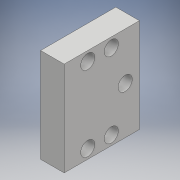
# Autodesk Inventor part: base_topPart
Saved by Autodesk Inventor 2018 (Build 220112000, 112)
## iProperties
Created: 2019-10-09
Part Number: base_topPart
Material: 一般
Document SubType Name: Modeling
Designer: Eiji Nishizawa
Density: 1 g/cm^3
Appearance: 既定
Author: Eiji Nishizawa
Autodesk Inventor part; units mm, degrees
ref_plane "YZ Plane" through (0, 0, 0) normal (1, 0, 0) x (0, 1, 0)
ref_plane "XZ Plane" through (0, 0, 0) normal (0, 1, 0) x (-1, 0, 0)
ref_plane "XY Plane" through (0, 0, 0) normal (0, 0, 1) x (1, 0, 0)
sketch "スケッチ1" plane through (0, 0, 0) normal (1, 0, 0) x (0, 1, 0)
  line L0 (-7.9816, 10) -> (7.9816, 10)
  line L1 (7.9816, 10) -> (7.9816, -10)
  line L2 (7.9816, -10) -> (-7.9816, -10)
  line L3 (-7.9816, -10) -> (-7.9816, 10)
  line L4 (-7.9816, 10) -> (7.9816, -10) construction
  line L5 (7.9816, 10) -> (-7.9816, -10) construction
  circle A0 centre (-2.9816, 8) radius 1.5
  circle A1 centre (2.0184, 8) radius 1.5
  circle A2 centre (2.0184, -8) radius 1.5
  circle A3 centre (-2.9816, -8) radius 1.5
  circle A4 centre (4.9684, 0) radius 1.5
  point P0 (0, 0)
  dimension "d0" = 3
  dimension "d1" = 3
  dimension "d2" = 3
  dimension "d3" = 3
  dimension "d4" = 5
  dimension "d5" = 5
  dimension "d6" = 20
  dimension "d7" = 16
  dimension "d8" = 2
  dimension "d9" = 2
  dimension "d10" = 5
  dimension "d11" = 2.95
  dimension "d12" = 3
  constraints: 12 end point, 5 centre point, 2 midpoint, 2 parallel, 1 horizontal, 1 perpendicular
  measures "d0" diameter of A1
  measures "d1" diameter of A0
  measures "d2" diameter of A3
  measures "d3" diameter of A2
  measures "d4" distance of A2.centre A3.centre
  measures "d5" distance of A1.centre A0.centre
  measures "d6" distance of L2.end L0.start
  measures "d7" distance of A3.centre A0.centre
  measures "d8" distance from line of L0 A0.centre
  measures "d9" distance from line of L2 A3.centre
  measures "d10" distance from line of L3 A0.centre
  measures "d11" horizontal distance of A4.centre A1.centre
  measures "d12" diameter of A4
extrude "押し出し1" add sketch "スケッチ1" along normal blind 5
